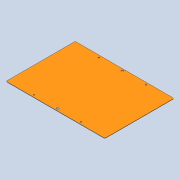
# Autodesk Inventor part: 14x20 ATNT Sign
Saved by Autodesk Inventor 2022 (Build 260153000, 153)
## iProperties
Created: 2022-01-01
Part Number: 14x20 ATNT Sign
Material: Generic
Document SubType Name: Modeling
Designer: Coy
Density: 1 g/cm^3
Appearance: Default
Author: Coy
Autodesk Inventor part; units mm, degrees
ref_plane "YZ Plane" through (0, 0, 0) normal (1, 0, 0) x (0, 1, 0)
ref_plane "XZ Plane" through (0, 0, 0) normal (0, 1, 0) x (-1, 0, 0)
ref_plane "XY Plane" through (0, 0, 0) normal (0, 0, 1) x (1, 0, 0)
sketch "Sketch1" plane through (0, 0, 0) normal (0, 1, 0) x (-1, 0, 0)
  line L0 (6.35, 0) -> (501.65, 0)
  line L1 (508, 6.35) -> (508, 349.25)
  line L2 (501.65, 355.6) -> (6.35, 355.6)
  line L3 (0, 349.25) -> (0, 6.35)
  line L4 (374.65, 344.4875) -> (133.35, 344.4875) construction
  line L5 (133.35, 344.4875) -> (133.35, 11.1125) construction
  line L6 (133.35, 11.1125) -> (374.65, 11.1125) construction
  line L7 (374.65, 11.1125) -> (374.65, 344.4875) construction
  line L8 (254, 344.4875) -> (254, 11.1125) construction
  line L9 (374.65, 344.4875) -> (508, 344.4875) construction
  line L10 (374.65, 344.4875) -> (374.65, 355.6) construction
  line L11 (133.35, 11.1125) -> (0, 11.1125) construction
  line L12 (133.35, 11.1125) -> (133.35, 0) construction
  circle A0 centre (374.65, 344.4875) radius 3.175
  circle A1 centre (374.65, 11.1125) radius 3.175
  circle A2 centre (133.35, 11.1125) radius 3.175
  circle A3 centre (133.35, 344.4875) radius 3.175
  circle A4 centre (254, 344.4875) radius 5.5562
  circle A5 centre (254, 11.1125) radius 5.5563
  arc A6 (508, 349.25) -> (501.65, 355.6) centre (501.65, 349.25) ccw
  arc A7 (501.65, 0) -> (508, 6.35) centre (501.65, 6.35) ccw
  arc A8 (0, 6.35) -> (6.35, 0) centre (6.35, 6.35) ccw
  arc A9 (6.35, 355.6) -> (0, 349.25) centre (6.35, 349.25) ccw
  point P0 (0, 0)
  point P1 (508, 355.6)
  point P2 (508, 0)
  point P3 (0, 355.6)
  dimension "d0" = 508
  dimension "d1" = 355.6
  dimension "d2" = 333.375
  dimension "d3" = 241.3
  dimension "d4" = 6.35
  dimension "d5" = 6.35
  dimension "d6" = 6.35
  dimension "d7" = 6.35
  dimension "d8" = 11.1125
  dimension "d9" = 11.1125
  dimension "d10" = 6.35
  constraints: 26 end point, 13 point on line, 10 centre point, 8 point on circle, 8 tangent, 6 coincident, 6 parallel, 5 perpendicular, 3 equal radius, 2 horizontal, 2 midpoint
  measures "d0" distance of point (0, 355.6) point (508, 355.6)
  measures "d1" distance of point (508, 355.6) point (508, 0)
  measures "d2" distance of L6.end L4.start
  measures "d3" distance of L4.start L4.end
  measures "d4" diameter of A0
  measures "d5" diameter of A1
  measures "d6" diameter of A2
  measures "d7" diameter of A3
  measures "d8" diameter of A4
  measures "d9" diameter of A5
  measures "d10" radius of A6
extrude "Extrusion1" add sketch "Sketch1" along normal blind 1.5875
equation "\"d5\" = d4"
equation "\"d6\" = d4"
equation "\"d7\" = d4"
equation "\"d9\" = d8"
body "Solid1"
